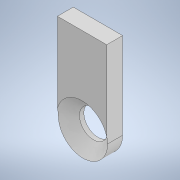
# Autodesk Inventor part: Part4
Saved by Autodesk Inventor 2022 (Build 260153000, 153)
## iProperties
Created: 2021-07-12
Part Number: Part4
Material: Generic
Document SubType Name: Modeling
Designer: Martijn
Density: 1 g/cm^3
Appearance: Default
Author: Martijn
Autodesk Inventor part; units mm, degrees
ref_plane "YZ Plane" through (0, 0, 0) normal (1, 0, 0) x (0, 1, 0)
ref_plane "XZ Plane" through (0, 0, 0) normal (0, 1, 0) x (-1, 0, 0)
ref_plane "XY Plane" through (0, 0, 0) normal (0, 0, 1) x (1, 0, 0)
sketch "Sketch1" plane through (0, 0, 0) normal (0, 0, 1) x (1, 0, 0)
  arc A0 (-2.8, 0) -> (2.8, 0) centre (0, 0) ccw
  circle A1 centre (0, 0) radius 1.6
  line L0 (-2.8, 0) -> (-2.8, 9.8)
  line L1 (-2.8, 9.8) -> (2.8, 9.8)
  line L2 (2.8, 9.8) -> (2.8, 0)
  dimension "d0" = 3.2
  dimension "d1" = 2.8
  dimension "d2" = 9.8
  constraints: 6 end point, 2 centre point, 2 coincident, 2 perpendicular, 2 point on circle, 2 tangent, 1 vertical
  measures "d0" diameter of A1
  measures "d1" radius of A0
  measures "d2" distance of L0.start L0.end
extrude "Extrusion1" add sketch "Sketch1" along normal blind 1.8
chamfer "Chamfer1" distance 1.3 angle 45 1 edges at (-1.6, 0, 1.8)
body "Solid1"
